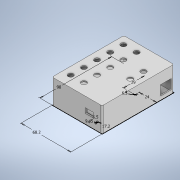
# Autodesk Inventor part: Part1
Saved by Autodesk Inventor 2020 (Build 240168000, 168)
## iProperties
Created: 2021-04-10
Part Number: Part1
Material: Generic
Document SubType Name: Modeling
Designer: Vlasciar
Density: 1 g/cm^3
Appearance: Default
Author: Vlasciar
Autodesk Inventor part; units mm, degrees
ref_plane "YZ Plane" through (0, 0, 0) normal (1, 0, 0) x (0, 1, 0)
ref_plane "XZ Plane" through (0, 0, 0) normal (0, 1, 0) x (-1, 0, 0)
ref_plane "XY Plane" through (0, 0, 0) normal (0, 0, 1) x (1, 0, 0)
sketch "Sketch1" plane through (0, 0, 0) normal (0, 1, 0) x (-1, 0, 0)
  line L0 (-34.1, -49) -> (34.1, -49)
  line L1 (34.1, -49) -> (34.1, 49)
  line L2 (34.1, 49) -> (-34.1, 49)
  line L3 (-34.1, 49) -> (-34.1, -49)
  line L4 (-34.1, -49) -> (34.1, 49) construction
  line L5 (34.1, -49) -> (-34.1, 49) construction
  circle A0 centre (-16.9, 39.55) radius 2
  circle A1 centre (-16.9, 39.55) radius 3.25
  line L6 (-18.8909, 27.1453) -> (-18.8909, 26.9568)
  circle A2 centre (-10.1, -20) radius 2
  circle A3 centre (-10.1, -20) radius 3.25
  point P0 (0, 0)
  dimension "d0" = 68.2
  dimension "d1" = 98
  dimension "d6" = 4
  dimension "d7" = 6.5
  dimension "d8" = 17.2
  dimension "d9" = 9.45
  dimension "d10" = 24
  dimension "d11" = 29
  dimension "d12" = 4
  dimension "d13" = 6.5
  constraints: 14 end point, 4 centre point, 4 coincident, 2 midpoint, 2 parallel, 2 perpendicular, 1 horizontal, 1 point on line
  measures "d0" distance of L1.end L2.end
  measures "d1" distance of L0.end L1.end
  measures "d6" diameter of A0
  measures "d7" diameter of A1
  measures "d8" distance from line of L3 A0.centre
  measures "d9" distance from line of L2 A0.centre
  measures "d10" distance from line of L3 point (-10.1, -20)
  measures "d11" distance from line of L0 point (-10.1, -20)
  measures "d12" diameter of A2
  measures "d13" diameter of A3
extrude "Extrusion1" add sketch "Sketch1" along normal blind 31.8 contours L3 L2 L1 L0 | A0 | A1 | A2 | A3
shell "Shell1" thickness 1.5 removed faces 1 at (11.3667, 31.8, 16.3333)
extrude "Extrusion2" add sketch "Sketch1" along normal blind 4.5 contours A1 | A3
sketch "Sketch2" plane through (-34.1, 0, 49) normal (0, 0, 1) x (1, 0, 0)
  line L0 (0, 0) -> (68.2, 0) projected
  line L1 (68.2, 0) -> (68.2, 31.8) projected
  line L2 (68.2, 0) -> (68.2, 31.8) projected
  line L3 (68.2, 1.5) -> (40, 1.5)
  line L4 (68, 6) -> (36, 6)
  line L5 (36, 6) -> (36, 4.5)
  line L6 (36, 4.5) -> (68, 4.5)
  line L7 (68, 4.5) -> (68, 6)
  line L8 (47.2, 17.65) -> (54.7, 17.65)
  line L9 (54.7, 17.65) -> (54.7, 14.9)
  line L10 (54.7, 14.9) -> (47.2, 14.9)
  line L11 (47.2, 14.9) -> (47.2, 17.65)
  line L12 (47.2, 17.65) -> (54.7, 14.9)
  line L13 (54.7, 17.65) -> (47.2, 14.9)
  line L14 (55.7, 13.9) -> (46.2, 13.9)
  line L15 (46.2, 13.9) -> (46.2, 18.65)
  line L16 (46.2, 18.65) -> (55.7, 18.65)
  line L17 (55.7, 18.65) -> (55.7, 13.9)
  line L18 (55.7, 13.9) -> (46.2, 18.65) construction
  line L19 (46.2, 13.9) -> (55.7, 18.65) construction
  point P0 (34.1, 0)
  point P1 (50.95, 16.275)
  dimension "d19" = 1.5
  dimension "d20" = 3
  dimension "d21" = 1.5
  dimension "d22" = 8.9
  dimension "d23" = 7.5
  dimension "d24" = 2.75
  dimension "d25" = 13.5
  dimension "d26" = 1
  dimension "d27" = 1
  constraints: 34 end point, 6 parallel, 4 horizontal, 3 midpoint, 3 perpendicular, 1 point on line
  measures "d19" distance between parallel lines of L0 L3
  measures "d20" distance between parallel lines of L3 L6
  measures "d21" distance between parallel lines of L4 L6
  measures "d22" distance between parallel lines of L4 L10
  measures "d23" distance between parallel lines of L9 L11
  measures "d24" distance between parallel lines of L8 L10
  measures "d25" distance between parallel lines of L1 L9
  measures "d26" distance between parallel lines of L11 L15
  measures "d27" distance between parallel lines of L16 L8
extrude "Extrusion3" cut sketch "Sketch2" against normal blind 4.5 contours L12 L13 L11 | L8 L13 L12 | L9 L12 L13 | L13 L12 L10 | L14 L15 L16 L17
fillet "Fillet1" radius 1 4 edges at (16.85, 18.65, 49) (21.6, 16.275, 49) (16.85, 13.9, 49) (12.1, 16.275, 49)
sketch "Sketch3" plane through (34.1, 0, 49) normal (1, 0, 0) x (0, 0, -1)
  line L0 (0, 0) -> (98, 0) projected
  line L1 (98, 0) -> (98, 31.8) projected
  line L2 (80.7, 17.4) -> (93.6, 17.4)
  line L3 (93.6, 17.4) -> (93.6, 6)
  line L4 (93.6, 6) -> (80.7, 6)
  line L5 (80.7, 6) -> (80.7, 17.4)
  line L6 (80.7, 17.4) -> (93.6, 6) construction
  line L7 (93.6, 17.4) -> (80.7, 6) construction
  line L8 (94.6, 5) -> (79.7, 5)
  line L9 (79.7, 5) -> (79.7, 18.4)
  line L10 (79.7, 18.4) -> (94.6, 18.4)
  line L11 (94.6, 18.4) -> (94.6, 5)
  line L12 (94.6, 5) -> (79.7, 18.4) construction
  line L13 (79.7, 5) -> (94.6, 18.4) construction
  point P0 (49, 0)
  point P1 (87.15, 11.7)
  point P2 (87.15, 11.7)
  dimension "d31" = 6
  dimension "d32" = 4.4
  dimension "d33" = 11.4
  dimension "d34" = 12.9
  dimension "d35" = 1
  dimension "d36" = 1
  constraints: 24 end point, 4 midpoint, 4 parallel, 2 horizontal, 2 perpendicular, 1 coincident
  measures "d31" distance between parallel lines of L0 L4
  measures "d32" distance between parallel lines of L1 L3
  measures "d33" distance between parallel lines of L2 L4
  measures "d34" distance between parallel lines of L5 L3
  measures "d35" distance between parallel lines of L5 L9
  measures "d36" distance between parallel lines of L10 L2
extrude "Extrusion4" cut sketch "Sketch3" against normal blind 4.5 contours L2 L3 L4 L5 | L8 L9 L10 L11
sketch "Sketch4" plane through (34.1, 0, -49) normal (0, 0, -1) x (-1, 0, 0)
  line L0 (0, 0) -> (68.2, 0) projected
  line L1 (0, 0) -> (0, 31.8) projected
  line L2 (28.8, 6) -> (20.1, 6)
  line L3 (20.1, 6) -> (20.1, 16.6)
  line L4 (20.1, 16.6) -> (28.8, 16.6)
  line L5 (28.8, 16.6) -> (28.8, 6)
  line L6 (28.8, 6) -> (20.1, 16.6) construction
  line L7 (20.1, 6) -> (28.8, 16.6) construction
  line L8 (29.8, 5) -> (19.1, 5)
  line L9 (19.1, 5) -> (19.1, 17.6)
  line L10 (19.1, 17.6) -> (29.8, 17.6)
  line L11 (29.8, 17.6) -> (29.8, 5)
  line L12 (29.8, 5) -> (19.1, 17.6) construction
  line L13 (19.1, 5) -> (29.8, 17.6) construction
  point P0 (34.1, 0)
  point P1 (24.45, 11.3)
  dimension "d39" = 20.1
  dimension "d40" = 6
  dimension "d41" = 8.7
  dimension "d42" = 10.6
  dimension "d43" = 1
  dimension "d44" = 1
  constraints: 24 end point, 4 midpoint, 4 parallel, 2 horizontal, 2 perpendicular
  measures "d39" distance between parallel lines of L1 L3
  measures "d40" distance between parallel lines of L0 L2
  measures "d41" distance of L2.start L2.end
  measures "d42" distance of L2.end L3.end
  measures "d43" distance between parallel lines of L10 L4
  measures "d44" distance between parallel lines of L9 L3
extrude "Extrusion5" cut sketch "Sketch4" against normal blind 4.5 contours L2 L3 L4 L5 | L8 L9 L10 L11
sketch "Sketch5" plane through (0, 31.8, 0) normal (0, 1, 0) x (1, 0, 0)
  line L0 (32.6, -47.5) -> (-32.6, -47.5) projected
  line L1 (-32.6, -47.5) -> (-32.6, 47.5) projected
  line L2 (-32.6, 47.5) -> (32.6, 47.5) projected
  line L3 (32.6, 47.5) -> (32.6, -47.5) projected
  line L4 (34.1, -49) -> (34.1, 49) projected
  line L5 (34.1, 49) -> (-34.1, 49) projected
  line L6 (-34.1, 49) -> (-34.1, -49) projected
  line L7 (-34.1, -49) -> (34.1, -49) projected
  line L8 (34.1, -49) -> (-34.1, -49)
  line L9 (-34.1, -49) -> (-34.1, 49)
  line L10 (-34.1, 49) -> (34.1, 49)
  line L11 (34.1, 49) -> (34.1, -49)
  circle A0 centre (-23.6, -34.15) radius 3
  circle A1 centre (-23.6, -34.15) radius 3.5
  circle A2 centre (-5.6, -34.15) radius 3.5
  circle A3 centre (-23.6, -16.15) radius 3.5
  circle A4 centre (-5.6, -16.15) radius 3.5
  circle A5 centre (-23.6, 1.85) radius 3.5
  circle A6 centre (-5.6, 1.85) radius 3.5
  circle A7 centre (-23.6, 19.85) radius 3.5
  circle A8 centre (-5.6, 19.85) radius 3.5
  circle A9 centre (-23.6, 37.85) radius 3.5
  circle A10 centre (-5.6, 37.85) radius 3.5
  circle A11 centre (-5.6, 1.85) radius 3.5
  circle A12 centre (21.9, 19.85) radius 3.5
  circle A13 centre (21.9, 1.85) radius 3.5
  line L12 (34.1, -49) -> (-34.1, -49)
  line L13 (-34.1, -49) -> (-34.1, 49)
  line L14 (-34.1, 49) -> (34.1, 49)
  line L15 (34.1, 49) -> (34.1, -49)
  point P0 (0, 0)
  dimension "d47" = 6
  dimension "d48" = 7
  dimension "d50" = 13.35
  dimension "d51" = 9
  dimension "d54" = 18
  dimension "d57" = 18
  dimension "d62" = 18
  dimension "d65" = 18
  dimension "d70" = 18
  dimension "d73" = 27.5
  constraints: 16 end point, 14 centre point, 5 horizontal, 4 parallel, 3 vertical, 2 perpendicular, 1 coincident, 33 other
  measures "d47" diameter of A0
  measures "d48" diameter of A1
  measures "d50" distance from line of L0 A0.centre
  measures "d51" distance from line of L1 A0.centre
  measures "d54" distance of A0.centre point (-5.6, -34.15)
  measures "d57" distance of A0.centre point (-23.6, -16.15)
  measures "d62" distance of A1.centre A2.centre
  measures "d65" distance of A1.centre A3.centre
  measures "d70" distance of A8.centre A11.centre
  measures "d73" distance of A8.centre A12.centre
extrude "Extrusion6" add sketch "Sketch5" along normal blind 1.5 contours L0 L1 L2 L3 | L7 L6 L5 L4
fillet "Fillet2" radius 2 4 edges at (34.1, 16.65, -49) (-34.1, 16.65, -49) (34.1, 16.65, 49) (-34.1, 16.65, 49)
body "Solid1"
